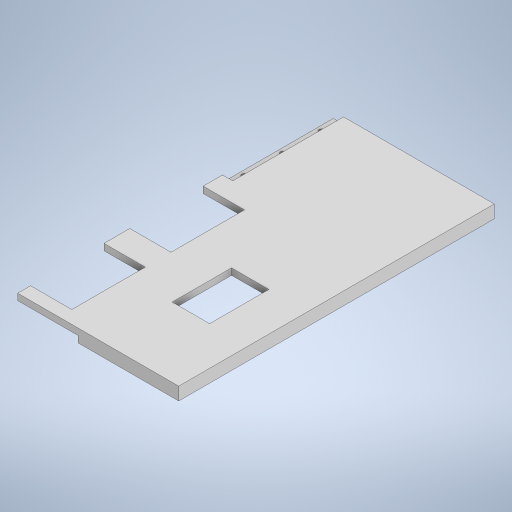
# Autodesk Inventor part: top_4
Saved by Autodesk Inventor 2023 (Build 270158000, 158)
## iProperties
Created: 2024-04-26
Part Number: top_4
Material: 常规
Document SubType Name: Modeling
Designer: Nitrene.P.L
Density: 1 g/cm^3
Appearance: 默认
Author: Nitrene.P.L
Autodesk Inventor part; units mm, degrees
ref_plane "YZ Plane" through (0, 0, 0) normal (1, 0, 0) x (0, 1, 0)
ref_plane "XZ Plane" through (0, 0, 0) normal (0, 1, 0) x (-1, 0, 0)
ref_plane "XY Plane" through (0, 0, 0) normal (0, 0, 1) x (1, 0, 0)
sketch "草图1" plane through (0, 0, 0) normal (0, 1, 0) x (-1, 0, 0)
  line L0 (-95, 54) -> (-66, 54)
  line L1 (-66, 54) -> (-66, 100)
  line L2 (-66, 100) -> (-95, 100)
  line L3 (-95, 100) -> (-95, 54)
  line L4 (-32, 144) -> (-32, 87)
  line L5 (-125, 0) -> (-125, 245)
  line L6 (-32, 87) -> (25, 87)
  line L7 (-125, 245) -> (-125, -245)
  line L8 (125, -245) -> (125, 245)
  line L9 (25, 144) -> (-32, 144)
  line L10 (-125, 245) -> (0, 245)
  line L11 (125, 245) -> (-125, 245)
  line L12 (25, 67) -> (-32, 67)
  line L13 (0, 0) -> (125, 0)
  line L14 (-32, 67) -> (-32, 10)
  line L15 (-32, 10) -> (25, 10)
  line L16 (3.5058, 0) -> (-3.4421, 0)
  line L17 (-66, -100) -> (-66, -54)
  line L18 (-95, -54) -> (-95, -100)
  line L19 (-95, -100) -> (-66, -100)
  line L20 (25, 87) -> (25, 144)
  line L21 (0, 245) -> (0, 0)
  line L22 (0, 245) -> (0, 0)
  line L23 (125, 0) -> (125, 245)
  line L24 (100, 15) -> (70, 15)
  line L25 (100, -15) -> (100, 15)
  line L26 (70, 15) -> (70, -15)
  line L27 (25, 10) -> (25, 67)
  line L28 (-125, -245) -> (125, -245)
  line L29 (-32, -87) -> (-32, -144)
  line L30 (-32, -10) -> (-32, -67)
  line L31 (25, -87) -> (-32, -87)
  line L32 (-32, -67) -> (25, -67)
  line L33 (25, -10) -> (-32, -10)
  line L34 (-32, -144) -> (25, -144)
  line L35 (-125, 0) -> (-125, -245)
  line L36 (25, -144) -> (25, -87)
  line L37 (25, -67) -> (25, -10)
  circle A0 centre (65, -182) radius 10
  line L38 (70, -15) -> (100, -15)
  line L39 (0, 0) -> (125, 0)
  line L40 (0, -245) -> (0, 0)
  line L41 (0, -245) -> (0, 0)
  line L42 (125, -245) -> (0, -245)
  line L43 (125, 0) -> (125, -245)
  line L44 (-125, -245) -> (0, -245)
  line L45 (0, 3) -> (0, -5)
  line L46 (-66, -54) -> (-95, -54)
  line L47 (0, 0) -> (-125, 0)
  line L48 (0, 0) -> (-125, 0)
  circle A1 centre (57.5, 194.9904) radius 1.5
  circle A2 centre (57.5, 169.0096) radius 1.5
  circle A3 centre (65, 182) radius 10
  circle A4 centre (65, 182) radius 15
  circle A5 centre (80, 182) radius 1.5
  line L49 (125, 245) -> (0, 245)
  circle A6 centre (65, -182) radius 15
  circle A7 centre (80, -182) radius 1.5
  circle A8 centre (57.5, -169.0096) radius 1.5
  circle A9 centre (57.5, -194.9904) radius 1.5
  point P0 (0, -10)
  point P1 (0, -144)
  point P2 (0, -87)
  point P3 (0, -67)
  dimension "d35" = 30
  dimension "d38" = 30
  dimension "d4" = 490
  dimension "d5" = 250
  dimension "d6" = 57
  dimension "d7" = 57
  dimension "d8" = 57
  dimension "d9" = 57
  dimension "d10" = 57
  dimension "d11" = 57
  dimension "d12" = 57
  dimension "d13" = 57
  dimension "d14" = 101
  dimension "d15" = 20
  dimension "d16" = 20
  dimension "d17" = 20
  dimension "d18" = 93
  dimension "d19" = 29
  dimension "d20" = 46
  dimension "d21" = 46
  dimension "d22" = 145
  dimension "d23" = 108
  dimension "d24" = 30
  dimension "d25" = 30
  dimension "d26" = 30
  dimension "d27" = 25
  dimension "d28" = 230
  dimension "d29" = 20
  dimension "d30" = 63
  dimension "d31" = 60
  dimension "d32" = 20
  dimension "d33" = 63
  dimension "d34" = 60
  dimension "d36" = 3
  dimension "d37" = 360
  dimension "d39" = 3
  dimension "d40" = 360
  constraints: 100 end point, 24 parallel, 14 horizontal, 12 perpendicular, 8 centre point, 3 collinear, 2 coincident, 2 horizontal alignment, 2 point on line, 2 vertical, 20 other
  measures "d4" distance of L43.end L8.end
  measures "d5" distance of L8.end L7.start
  measures "d6" distance of L6.end L4.end
  measures "d7" distance of L4.end L4.start
  measures "d8" distance of L15.end L15.start
  measures "d9" distance of L15.start L12.end
  measures "d10" distance of L37.start L32.start
  measures "d11" distance of L32.start L33.end
  measures "d12" distance of L34.end L34.start
  measures "d13" distance of L34.start L31.end
  measures "d14" distance between parallel lines of L11 L9
  measures "d15" distance between parallel lines of L12 L6
  measures "d16" distance between parallel lines of L15 L33
  measures "d17" distance between parallel lines of L31 L32
  measures "d18" distance between parallel lines of L7 L4
  measures "d19" distance of L0.end L0.start
  measures "d20" distance of L0.start L2.end
  measures "d21" distance of L18.end L18.start
  measures "d22" distance between parallel lines of L11 L2
  measures "d23" distance between parallel lines of L46 L0
  measures "d24" distance between parallel lines of L7 L3
  measures "d25" distance of L25.start L26.end
  measures "d26" distance of L26.end L24.end
  measures "d27" distance between parallel lines of L8 L25
  measures "d28" distance between parallel lines of L11 L24
  measures "d29" diameter of A3
  measures "d30" distance from line of L11 A3.centre
  measures "d31" distance from line of L8 A3.centre
  measures "d32" diameter of A0
  measures "d33" distance from line of L28 A0.centre
  measures "d34" distance from line of L8 A0.centre
  measures "d36" diameter of A5
  measures "d39" diameter of A7
extrude "拉伸1" add sketch "草图1" along normal blind 10 contours L47 L16 L40 L33 L30 L32 L31 L29 L34 L28 L7
sketch "草图2" plane through (0, 0, 0) normal (0, -1, 0) x (1, 0, 0)
  line L0 (110, -39) -> (47, -39)
  line L1 (47, -39) -> (47, -115)
  line L2 (47, -115) -> (110, -115)
  line L3 (110, -115) -> (110, -39)
  line L4 (95, -100) -> (95, -54) projected
  line L5 (66, -100) -> (95, -100) projected
  line L6 (95, -54) -> (66, -54) projected
  line L7 (66, -54) -> (66, -100) projected
  line L8 (0, 0) -> (125, 0) projected
  line L9 (47, 0) -> (0, 0)
  line L10 (0, 0) -> (0, -159)
  line L11 (0, -159) -> (47, -159)
  line L12 (47, -159) -> (47, 0)
  line L13 (32, -67) -> (32, -10) projected
  line L14 (0, -144) -> (32, -144) projected
  dimension "d43" = 15
  dimension "d44" = 15
  dimension "d45" = 15
  dimension "d46" = 19
  dimension "d47" = 15
  dimension "d48" = 15
  constraints: 16 end point, 4 parallel, 2 horizontal, 2 perpendicular, 1 point on line
  measures "d43" distance between parallel lines of L3 L4
  measures "d44" distance between parallel lines of L2 L5
  measures "d45" distance between parallel lines of L0 L6
  measures "d46" distance between parallel lines of L1 L7
  measures "d47" distance between parallel lines of L12 L13
  measures "d48" distance between parallel lines of L11 L14
extrude "拉伸2" cut sketch "草图2" against normal blind 5
sketch "草图3" plane through (0, 10, 0) normal (0, 1, 0) x (1, 0, 0)
  line L0 (0, 245) -> (8, 245)
  line L1 (8, 144) -> (0, 144)
  line L2 (125, 245) -> (0, 245) projected
  line L3 (47, 159) -> (0, 159) projected
  line L4 (0, 245) -> (8, 245)
  line L5 (8, 245) -> (8, 159)
  line L6 (8, 159) -> (0, 159)
  line L7 (0, 159) -> (0, 245)
  point P0 (0, 0)
  point P1 (0, 159)
  dimension "d65" = 8
  constraints: 12 end point, 3 parallel, 2 horizontal, 1 perpendicular, 1 point on line
  measures "d65" distance of L5.end L6.end
extrude "拉伸5" cut sketch "草图3" against normal blind 5
sketch "草图6" plane through (0, 5, 0) normal (0, 1, 0) x (1, 0, 0)
  circle A0 centre (4, 172) radius 2
  circle A1 centre (4, 202) radius 2
  circle A2 centre (4, 232) radius 2
  line L0 (8, 245) -> (8, 159) projected
  line L1 (8, 159) -> (0, 159) projected
  point P0 (0, 0)
  dimension "d68" = 4
  dimension "d69" = 4
  dimension "d70" = 4
  dimension "d71" = 4
  dimension "d72" = 4
  dimension "d73" = 4
  dimension "d74" = 13
  dimension "d75" = 30
  dimension "d76" = 30
  constraints: 3 centre point
  measures "d68" diameter of A0
  measures "d69" diameter of A1
  measures "d70" diameter of A2
  measures "d71" distance from line of L0 A0.centre
  measures "d72" distance from line of L0 A1.centre
  measures "d73" distance from line of L0 A2.centre
  measures "d74" distance from line of L1 A0.centre
  measures "d75" distance of A1.centre A0.centre
  measures "d76" distance of A2.centre A1.centre
extrude "拉伸6" cut sketch "草图6" against normal blind 5
